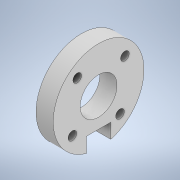
# Autodesk Inventor part: MotorMount
Saved by Autodesk Inventor 2022 (Build 260153000, 153)
## iProperties
Created: 2022-02-05
Part Number: MotorMount
Material: Generic
Document SubType Name: Modeling
Designer: ultra
Density: 1 g/cm^3
Appearance: Default
Author: ultra
Autodesk Inventor part; units mm, degrees
ref_plane "YZ Plane" through (0, 0, 0) normal (1, 0, 0) x (0, 1, 0)
ref_plane "XZ Plane" through (0, 0, 0) normal (0, 1, 0) x (-1, 0, 0)
ref_plane "XY Plane" through (0, 0, 0) normal (0, 0, 1) x (1, 0, 0)
sketch "Sketch1" plane through (0, 0, 0) normal (1, 0, 0) x (0, 1, 0)
  arc A0 (-16.1342, -4.5) -> (-16.1342, 4.5) centre (0, 0) ccw
  line L0 (-10.6472, 4.5) -> (-16.1342, 4.5)
  line L1 (-10.6472, -4.5) -> (-10.6472, 4.5)
  line L2 (-16.1342, -4.5) -> (-10.6472, -4.5)
  circle A1 centre (9.6916, 7.8945) radius 1.5
  circle A2 centre (7.8945, -9.6916) radius 1.5
  circle A3 centre (-9.6916, -7.8945) radius 1.5
  circle A4 centre (-7.8945, 9.6916) radius 1.5
  circle A5 centre (0, 0) radius 6.8
  circle A6 centre (9.6916, 7.8945) radius 1.5875
  circle A7 centre (7.8945, -9.6916) radius 1.5875
  circle A8 centre (-9.6916, -7.8945) radius 1.5875
  circle A9 centre (-7.8945, 9.6916) radius 1.5875
  dimension "d2" = 3.175
  dimension "d3" = 3.175
  dimension "d4" = 3.175
  dimension "d5" = 3.175
  constraints: 10 centre point, 6 end point, 4 coincident, 2 point on circle
  measures "d2" diameter of A6
  measures "d3" diameter of A7
  measures "d4" diameter of A8
  measures "d5" diameter of A9
extrude "Extrusion2" add sketch "Sketch1" along normal blind 6.35 contours L2 L1 L0 A0
body "Solid2"
